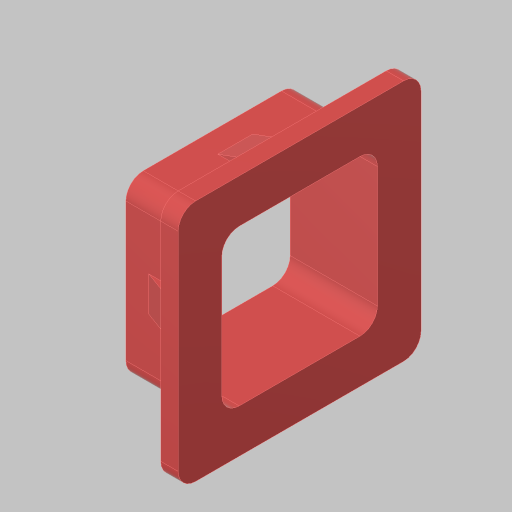
# Autodesk Inventor part: DB1-013
Saved by Autodesk Inventor 2023.5 (Build 275446000, 446)
## iProperties
Created: 2025-02-07
Part Number: DB1-013
Material: ABS Plastic
Document SubType Name: Modeling
Designer: slick
Density: 1.06 g/cm^3
Appearance: Smooth - Red
Author: slick
Autodesk Inventor part; units mm, degrees
ref_plane "YZ Plane" through (0, 0, 0) normal (1, 0, 0) x (0, 1, 0)
ref_plane "XZ Plane" through (0, 0, 0) normal (0, 1, 0) x (-1, 0, 0)
ref_plane "XY Plane" through (0, 0, 0) normal (0, 0, 1) x (1, 0, 0)
sketch "Sketch1" plane through (0, 0, 0) normal (1, 0, 0) x (0, 1, 0)
  line L0 (-15.748, -15.748) -> (15.748, -15.748)
  line L1 (15.748, -15.748) -> (15.748, 15.748)
  line L2 (15.748, 15.748) -> (-15.748, 15.748)
  line L3 (-15.748, 15.748) -> (-15.748, -15.748)
  line L4 (-15.748, -15.748) -> (15.748, 15.748) construction
  line L5 (15.748, -15.748) -> (-15.748, 15.748) construction
  line L6 (14.1605, 14.1605) -> (14.1605, -14.1605)
  line L7 (14.1605, -14.1605) -> (-14.1605, -14.1605)
  line L8 (-14.1605, -14.1605) -> (-14.1605, 14.1605)
  line L9 (-14.1605, 14.1605) -> (14.1605, 14.1605)
  point P0 (0, 0)
  dimension "d0" = 31.496
  dimension "d1" = 31.496
  dimension "d2" = 1.5875
  constraints: 20 end point, 4 parallel, 2 midpoint, 2 perpendicular, 1 horizontal, 3 other
  measures "d0" distance of L2.end L1.end
  measures "d1" distance between parallel lines of L0 L2
  measures "d2" distance between parallel lines of L1 L6
extrude "Extrusion1" add sketch "Sketch1" along normal blind 12.7
sketch "Sketch2" plane through (12.7, 0, 0) normal (1, 0, 0) x (0, 0, -1)
  line L0 (15.748, 15.748) -> (-15.748, 15.748) projected
  line L1 (-15.748, 15.748) -> (-15.748, -15.748) projected
  line L2 (-15.748, -15.748) -> (15.748, -15.748) projected
  line L3 (15.748, -15.748) -> (15.748, 15.748) projected
  line L4 (-14.1605, 14.1605) -> (14.1605, 14.1605) projected
  line L5 (14.1605, 14.1605) -> (14.1605, -14.1605) projected
  line L6 (14.1605, -14.1605) -> (-14.1605, -14.1605) projected
  line L7 (-14.1605, -14.1605) -> (-14.1605, 14.1605) projected
  line L8 (-22.098, 22.098) -> (22.098, 22.098)
  line L9 (22.098, 22.098) -> (22.098, -22.098)
  line L10 (22.098, -22.098) -> (-22.098, -22.098)
  line L11 (-22.098, -22.098) -> (-22.098, 22.098)
  point P0 (0, 0)
  dimension "d5" = 6.35
  constraints: 8 end point, 3 other
  measures "d5" distance between parallel lines of L0 L8
extrude "Extrusion2" add sketch "Sketch2" along normal blind 3.175 contours L3 L2 L1 L0 | L8 L9 L10 L11
fillet "Fillet1" radius 3.175 12 edges at (6.35, 15.748, 15.748) (6.35, 15.748, -15.748) (6.35, -15.748, 15.748) (6.35, -15.748, -15.748) (7.9375, 14.1605, 14.1605) (7.9375, -14.1605, 14.1605) (7.9375, -14.1605, -14.1605) (7.9375, 14.1605, -14.1605) (14.2875, -22.098, 22.098) (14.2875, -22.098, -22.098) (14.2875, 22.098, -22.098) (14.2875, 22.098, 22.098)
sketch "Sketch4" plane through (0, 0, 0) normal (0, 0, 1) x (1, 0, 0)
  line L0 (0, -15.748) -> (12.7, -15.748) construction
  line L1 (4.1641, -15.748) -> (9.398, -17.653)
  line L2 (9.398, -17.653) -> (9.398, -15.748)
  line L3 (12.7, -18.923) -> (12.7, 18.923) construction
  line L4 (4.1641, -15.748) -> (9.398, -15.748)
  point P0 (0, 0)
  dimension "d9" = 3.302
  dimension "d10" = 1.905
  dimension "d11" = 20
  constraints: 6 end point, 2 point on line, 1 collinear, 1 vertical
  measures "d9" distance between parallel lines of L3 L2
  measures "d10" distance from line of L0 L1.end
  measures "d11" angle of L0 L1
extrude "Extrusion3" add sketch "Sketch4" along normal mid plane 6.35
pattern_circular "Circular Pattern1" count 4 over 360 about axis through (-10, 0, 0) along (1, 0, 0) of "Extrusion3"
body "Solid1"
